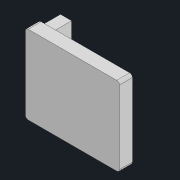
# Autodesk Inventor part: base_link
Saved by Autodesk Inventor 2021 (Build 250183000, 183)
## iProperties
Created: 2021-07-10
Part Number: base_link
Material: 一般
Document SubType Name: Modeling
Designer: yuta0
Density: 1 g/cm^3
Appearance: 既定
Author: yuta0
Autodesk Inventor part; units mm, degrees
ref_plane "YZ Plane" through (0, 0, 0) normal (1, 0, 0) x (0, 1, 0)
ref_plane "XZ Plane" through (0, 0, 0) normal (0, 1, 0) x (-1, 0, 0)
ref_plane "XY Plane" through (0, 0, 0) normal (0, 0, 1) x (1, 0, 0)
sketch "スケッチ1" plane through (0, 0, 0) normal (0, 0, 1) x (1, 0, 0)
  line L0 (-85, -71) -> (85, -71)
  line L1 (85, -71) -> (85, 71)
  line L2 (85, 71) -> (-85, 71)
  line L3 (-85, 71) -> (-85, -71)
  line L4 (-85, -71) -> (85, 71) construction
  line L5 (85, -71) -> (-85, 71) construction
  point P0 (0, 0)
  dimension "d0" = 170
  dimension "d1" = 142
  constraints: 12 end point, 2 midpoint, 2 parallel, 1 horizontal, 1 perpendicular
  measures "d0" distance of L1.end L2.end
  measures "d1" distance of L0.end L1.end
extrude "押し出し1" add sketch "スケッチ1" along normal blind 23.35
fillet "フィレット1" radius 5 4 edges at (-85, 71, 11.675) (-85, -71, 11.675) (85, 71, 11.675) (85, -71, 11.675)
sketch "スケッチ2" plane through (0, 0, 0) normal (0, 0, 1) x (1, 0, 0)
  arc A0 (80, -71) -> (85, -66) centre (80, -66) ccw projected
  line L0 (85, -66) -> (85, 66) projected
  arc A1 (85, 66) -> (80, 71) centre (80, 66) ccw projected
  line L1 (80, 71) -> (-80, 71) projected
  arc A2 (-80, 71) -> (-85, 66) centre (-80, 66) ccw projected
  line L2 (-85, 66) -> (-85, -66) projected
  arc A3 (-85, -66) -> (-80, -71) centre (-80, -66) ccw projected
  line L3 (-80, -71) -> (80, -71) projected
  line L4 (-60, 51) -> (60, 51)
  line L5 (60, 51) -> (60, 71)
  line L6 (60, 71) -> (-60, 71)
  line L7 (-60, 71) -> (-60, 51)
  line L8 (-60, 51) -> (60, 71) construction
  line L9 (60, 51) -> (-60, 71) construction
  line L10 (80, 71) -> (-80, 71) projected
  line L11 (-20, 71) -> (-20, 51)
  line L12 (20, 51) -> (20, 71)
  line L13 (-65, 60) -> (-85, 60)
  line L14 (-85, 60) -> (-85, -60)
  line L15 (-85, -60) -> (-65, -60)
  line L16 (-65, -60) -> (-65, 60)
  line L17 (-65, 60) -> (-85, -60) construction
  line L18 (-85, 60) -> (-65, -60) construction
  point P0 (0, 0)
  point P1 (0, 61)
  point P2 (0, 61)
  point P3 (-75, 0)
  point P4 (-75, 0)
  dimension "d5" = 120
  dimension "d6" = 20
  dimension "d9" = 40
  dimension "d10" = 40
  dimension "d11" = 120
  dimension "d12" = 20
  constraints: 28 end point, 6 midpoint, 6 point on line, 4 parallel, 4 perpendicular, 2 horizontal, 1 horizontal alignment, 1 vertical alignment
  measures "d5" distance of L5.end L6.end
  measures "d6" distance of L6.end L4.start
  measures "d9" distance between parallel lines of L7 L11
  measures "d10" distance between parallel lines of L5 L12
  measures "d11" distance of L15.end L13.start
  measures "d12" distance of L14.end L15.end
extrude "押し出し2" add sketch "スケッチ2" against normal blind 40 contours L2 L13 L16 L15
